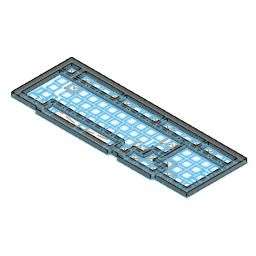
gotta crank v1 (Autodesk Fusion 360 design; units mm, degrees)
Autodesk Fusion 360 part; units mm, degrees
(part 1 of 2)
sketch "plate-2023-07-14T19_23_39.336Z" plane through (0, 0, 0) normal (0, 0, 1) x (1, 0, 0) in component "for my desk"
  arc A0 (50.65, -2.525) -> (50.15, -3.025) centre (50.65, -3.025) ccw
  line L0 (31.1, -3.025) -> (31.1, -16.025)
  line L1 (69.7, -2.525) -> (82.7, -2.525)
  arc A1 (125.5625, -16.525) -> (126.0625, -16.025) centre (125.5625, -16.025) ccw
  line L2 (131.6125, -2.525) -> (144.6125, -2.525)
  line L3 (112.0625, -3.025) -> (112.0625, -16.025)
  line L4 (131.1125, -3.025) -> (131.1125, -16.025)
  arc A2 (82.7, -16.525) -> (83.2, -16.025) centre (82.7, -16.025) ccw
  line L5 (50.65, -16.525) -> (63.65, -16.525)
  arc A3 (101.75, -16.525) -> (102.25, -16.025) centre (101.75, -16.025) ccw
  line L6 (88.25, -3.025) -> (88.25, -16.025)
  line L7 (131.6125, -16.525) -> (144.6125, -16.525)
  line L8 (145.1125, -3.025) -> (145.1125, -16.025)
  arc A4 (145.1125, -3.025) -> (144.6125, -2.525) centre (144.6125, -3.025) ccw
  arc A5 (144.6125, -16.525) -> (145.1125, -16.025) centre (144.6125, -16.025) ccw
  line L9 (150.6625, -16.525) -> (163.6625, -16.525)
  arc A6 (131.1125, -16.025) -> (131.6125, -16.525) centre (131.6125, -16.025) ccw
  arc A7 (150.6625, -2.525) -> (150.1625, -3.025) centre (150.6625, -3.025) ccw
  arc A8 (3.025, -2.525) -> (2.525, -3.025) centre (3.025, -3.025) ccw
  arc A9 (88.25, -16.025) -> (88.75, -16.525) centre (88.75, -16.025) ccw
  arc A10 (63.65, -16.525) -> (64.15, -16.025) centre (63.65, -16.025) ccw
  line L10 (69.2, -3.025) -> (69.2, -16.025)
  arc A11 (64.15, -3.025) -> (63.65, -2.525) centre (63.65, -3.025) ccw
  arc A12 (69.7, -2.525) -> (69.2, -3.025) centre (69.7, -3.025) ccw
  line L11 (126.0625, -3.025) -> (126.0625, -16.025)
  arc A13 (112.0625, -16.025) -> (112.5625, -16.525) centre (112.5625, -16.025) ccw
  arc A14 (131.6125, -2.525) -> (131.1125, -3.025) centre (131.6125, -3.025) ccw
  arc A15 (16.025, -16.525) -> (16.525, -16.025) centre (16.025, -16.025) ccw
  line L12 (150.1625, -3.025) -> (150.1625, -16.025)
  line L13 (31.6, -2.525) -> (44.6, -2.525)
  line L14 (88.75, -2.525) -> (101.75, -2.525)
  arc A16 (44.6, -16.525) -> (45.1, -16.025) centre (44.6, -16.025) ccw
  arc A17 (88.75, -2.525) -> (88.25, -3.025) centre (88.75, -3.025) ccw
  line L15 (50.65, -2.525) -> (63.65, -2.525)
  arc A18 (102.25, -3.025) -> (101.75, -2.525) centre (101.75, -3.025) ccw
  line L16 (112.5625, -16.525) -> (125.5625, -16.525)
  arc A19 (112.5625, -2.525) -> (112.0625, -3.025) centre (112.5625, -3.025) ccw
  arc A20 (126.0625, -3.025) -> (125.5625, -2.525) centre (125.5625, -3.025) ccw
  line L17 (102.25, -3.025) -> (102.25, -16.025)
  arc A21 (163.6625, -16.525) -> (164.1625, -16.025) centre (163.6625, -16.025) ccw
  arc A22 (250.175, -16.025) -> (250.675, -16.525) centre (250.675, -16.025) ccw
  line L18 (250.675, -16.525) -> (263.675, -16.525)
  line L19 (307.0375, -3.025) -> (307.0375, -16.025)
  line L20 (250.175, -3.025) -> (250.175, -16.025)
  line L21 (212.075, -3.025) -> (212.075, -16.025)
  arc A23 (293.0375, -16.025) -> (293.5375, -16.525) centre (293.5375, -16.025) ccw
  line L22 (312.5875, -2.525) -> (325.5875, -2.525)
  line L23 (312.0875, -3.025) -> (312.0875, -16.025)
  arc A24 (206.525, -16.525) -> (207.025, -16.025) centre (206.525, -16.025) ccw
  line L24 (245.125, -3.025) -> (245.125, -16.025)
  line L25 (212.575, -2.525) -> (225.575, -2.525)
  line L26 (287.9875, -3.025) -> (287.9875, -16.025)
  line L27 (169.7125, -2.525) -> (182.7125, -2.525)
  line L28 (2.525, -3.025) -> (2.525, -16.025)
  line L29 (274.4875, -16.525) -> (287.4875, -16.525)
  arc A25 (225.575, -16.525) -> (226.075, -16.025) centre (225.575, -16.025) ccw
  arc A26 (2.525, -16.025) -> (3.025, -16.525) centre (3.025, -16.025) ccw
  line L30 (193.525, -16.525) -> (206.525, -16.525)
  arc A27 (182.7125, -16.525) -> (183.2125, -16.025) centre (182.7125, -16.025) ccw
  line L31 (193.525, -2.525) -> (206.525, -2.525)
  line L32 (183.2125, -3.025) -> (183.2125, -16.025)
  line L33 (231.625, -16.525) -> (244.625, -16.525)
  arc A28 (264.175, -3.025) -> (263.675, -2.525) centre (263.675, -3.025) ccw
  arc A29 (287.4875, -16.525) -> (287.9875, -16.025) centre (287.4875, -16.025) ccw
  arc A30 (245.125, -3.025) -> (244.625, -2.525) centre (244.625, -3.025) ccw
  arc A31 (183.2125, -3.025) -> (182.7125, -2.525) centre (182.7125, -3.025) ccw
  line L34 (69.7, -16.525) -> (82.7, -16.525)
  arc A32 (31.6, -2.525) -> (31.1, -3.025) centre (31.6, -3.025) ccw
  line L35 (231.625, -2.525) -> (244.625, -2.525)
  line L36 (264.175, -3.025) -> (264.175, -16.025)
  line L37 (207.025, -3.025) -> (207.025, -16.025)
  line L38 (293.5375, -2.525) -> (306.5375, -2.525)
  arc A33 (274.4875, -2.525) -> (273.9875, -3.025) centre (274.4875, -3.025) ccw
  arc A34 (212.575, -2.525) -> (212.075, -3.025) centre (212.575, -3.025) ccw
  arc A35 (306.5375, -16.525) -> (307.0375, -16.025) centre (306.5375, -16.025) ccw
  arc A36 (164.1625, -3.025) -> (163.6625, -2.525) centre (163.6625, -3.025) ccw
  arc A37 (193.525, -2.525) -> (193.025, -3.025) centre (193.525, -3.025) ccw
  line L39 (226.075, -3.025) -> (226.075, -16.025)
  arc A38 (307.0375, -3.025) -> (306.5375, -2.525) centre (306.5375, -3.025) ccw
  line L40 (293.5375, -16.525) -> (306.5375, -16.525)
  arc A39 (273.9875, -16.025) -> (274.4875, -16.525) centre (274.4875, -16.025) ccw
  arc A40 (169.2125, -16.025) -> (169.7125, -16.525) centre (169.7125, -16.025) ccw
  arc A41 (150.1625, -16.025) -> (150.6625, -16.525) centre (150.6625, -16.025) ccw
  line L41 (169.2125, -3.025) -> (169.2125, -16.025)
  line L42 (293.0375, -3.025) -> (293.0375, -16.025)
  line L43 (212.575, -16.525) -> (225.575, -16.525)
  arc A42 (287.9875, -3.025) -> (287.4875, -2.525) centre (287.4875, -3.025) ccw
  arc A43 (293.5375, -2.525) -> (293.0375, -3.025) centre (293.5375, -3.025) ccw
  arc A44 (250.675, -2.525) -> (250.175, -3.025) centre (250.675, -3.025) ccw
  arc A45 (120.8, -40.3375) -> (121.3, -39.8375) centre (120.8, -39.8375) ccw
  arc A46 (63.65, -40.3375) -> (64.15, -39.8375) centre (63.65, -39.8375) ccw
  arc A47 (107.8, -26.3375) -> (107.3, -26.8375) centre (107.8, -26.8375) ccw
  arc A48 (244.625, -16.525) -> (245.125, -16.025) centre (244.625, -16.025) ccw
  line L44 (45.1, -26.8375) -> (45.1, -39.8375)
  line L45 (7.2875, -26.8375) -> (7.2875, -39.8375)
  line L46 (69.2, -26.8375) -> (69.2, -39.8375)
  arc A49 (325.5875, -16.525) -> (326.0875, -16.025) centre (325.5875, -16.025) ccw
  arc A50 (312.5875, -2.525) -> (312.0875, -3.025) centre (312.5875, -3.025) ccw
  line L47 (7.7875, -40.3375) -> (20.7875, -40.3375)
  line L48 (31.1, -26.8375) -> (31.1, -39.8375)
  line L49 (145.9, -26.3375) -> (158.9, -26.3375)
  line L50 (145.9, -40.3375) -> (158.9, -40.3375)
  line L51 (145.4, -26.8375) -> (145.4, -39.8375)
  arc A51 (169.7125, -2.525) -> (169.2125, -3.025) centre (169.7125, -3.025) ccw
  line L52 (21.2875, -26.8375) -> (21.2875, -39.8375)
  arc A52 (207.025, -3.025) -> (206.525, -2.525) centre (206.525, -3.025) ccw
  line L53 (50.15, -26.8375) -> (50.15, -39.8375)
  arc A53 (44.6, -40.3375) -> (45.1, -39.8375) centre (44.6, -39.8375) ccw
  line L54 (159.4, -26.8375) -> (159.4, -39.8375)
  arc A54 (126.35, -39.8375) -> (126.85, -40.3375) centre (126.85, -39.8375) ccw
  arc A55 (7.2875, -39.8375) -> (7.7875, -40.3375) centre (7.7875, -39.8375) ccw
  line L55 (64.15, -26.8375) -> (64.15, -39.8375)
  line L56 (273.9875, -3.025) -> (273.9875, -16.025)
  arc A56 (31.6, -26.3375) -> (31.1, -26.8375) centre (31.6, -26.8375) ccw
  arc A57 (88.25, -39.8375) -> (88.75, -40.3375) centre (88.75, -39.8375) ccw
  line L57 (126.35, -26.8375) -> (126.35, -39.8375)
  line L58 (121.3, -26.8375) -> (121.3, -39.8375)
  line L59 (126.85, -26.3375) -> (139.85, -26.3375)
  line L60 (107.8, -26.3375) -> (120.8, -26.3375)
  line L61 (326.0875, -3.025) -> (326.0875, -16.025)
  line L62 (312.5875, -16.525) -> (325.5875, -16.525)
  arc A58 (88.75, -26.3375) -> (88.25, -26.8375) centre (88.75, -26.8375) ccw
  arc A59 (50.15, -39.8375) -> (50.65, -40.3375) centre (50.65, -39.8375) ccw
  arc A60 (69.7, -26.3375) -> (69.2, -26.8375) centre (69.7, -26.8375) ccw
  arc A61 (193.025, -16.025) -> (193.525, -16.525) centre (193.525, -16.025) ccw
  line L63 (140.35, -26.8375) -> (140.35, -39.8375)
  arc A62 (82.7, -40.3375) -> (83.2, -39.8375) centre (82.7, -39.8375) ccw
  line L64 (102.25, -26.8375) -> (102.25, -39.8375)
  arc A63 (101.75, -40.3375) -> (102.25, -39.8375) centre (101.75, -39.8375) ccw
  line L65 (83.2, -26.8375) -> (83.2, -39.8375)
  arc A64 (139.85, -40.3375) -> (140.35, -39.8375) centre (139.85, -39.8375) ccw
  arc A65 (107.3, -39.8375) -> (107.8, -40.3375) centre (107.8, -39.8375) ccw
  arc A66 (20.7875, -40.3375) -> (21.2875, -39.8375) centre (20.7875, -39.8375) ccw
  line L66 (274.4875, -2.525) -> (287.4875, -2.525)
  line L67 (88.75, -40.3375) -> (101.75, -40.3375)
  arc A67 (83.2, -26.8375) -> (82.7, -26.3375) centre (82.7, -26.8375) ccw
  line L68 (250.675, -2.525) -> (263.675, -2.525)
  line L69 (193.025, -3.025) -> (193.025, -16.025)
  arc A68 (212.075, -16.025) -> (212.575, -16.525) centre (212.575, -16.025) ccw
  line L70 (69.7, -26.3375) -> (82.7, -26.3375)
  arc A69 (145.9, -26.3375) -> (145.4, -26.8375) centre (145.9, -26.8375) ccw
  arc A70 (231.625, -2.525) -> (231.125, -3.025) centre (231.625, -3.025) ccw
  line L71 (169.7125, -16.525) -> (182.7125, -16.525)
  arc A71 (226.075, -3.025) -> (225.575, -2.525) centre (225.575, -3.025) ccw
  arc A72 (21.2875, -26.8375) -> (20.7875, -26.3375) centre (20.7875, -26.8375) ccw
  line L72 (231.125, -3.025) -> (231.125, -16.025)
  arc A73 (231.125, -16.025) -> (231.625, -16.525) centre (231.625, -16.025) ccw
  arc A74 (263.675, -16.525) -> (264.175, -16.025) centre (263.675, -16.025) ccw
  arc A75 (69.2, -39.8375) -> (69.7, -40.3375) centre (69.7, -39.8375) ccw
  arc A76 (64.15, -26.8375) -> (63.65, -26.3375) centre (63.65, -26.8375) ccw
  arc A77 (140.35, -26.8375) -> (139.85, -26.3375) centre (139.85, -26.8375) ccw
  line L73 (107.8, -40.3375) -> (120.8, -40.3375)
  arc A78 (121.3, -26.8375) -> (120.8, -26.3375) centre (120.8, -26.8375) ccw
  arc A79 (287.4875, -40.3375) -> (287.9875, -39.8375) centre (287.4875, -39.8375) ccw
  arc A80 (273.9875, -39.8375) -> (274.4875, -40.3375) centre (274.4875, -39.8375) ccw
  line L74 (293.5375, -40.3375) -> (306.5375, -40.3375)
  arc A81 (164.45, -39.8375) -> (164.95, -40.3375) centre (164.95, -39.8375) ccw
  arc A82 (45.1, -26.8375) -> (44.6, -26.3375) centre (44.6, -26.8375) ccw
  line L75 (255.4375, -40.3375) -> (268.4375, -40.3375)
  line L76 (202.55, -26.8375) -> (202.55, -39.8375)
  arc A83 (216.55, -26.8375) -> (216.05, -26.3375) centre (216.05, -26.8375) ccw
  arc A84 (197.5, -26.8375) -> (197, -26.3375) centre (197, -26.8375) ccw
  arc A85 (184, -26.3375) -> (183.5, -26.8375) centre (184, -26.8375) ccw
  line L77 (184, -40.3375) -> (197, -40.3375)
  arc A86 (293.0375, -39.8375) -> (293.5375, -40.3375) centre (293.5375, -39.8375) ccw
  line L78 (274.4875, -40.3375) -> (287.4875, -40.3375)
  arc A87 (268.9375, -26.8375) -> (268.4375, -26.3375) centre (268.4375, -26.8375) ccw
  line L79 (88.75, -26.3375) -> (101.75, -26.3375)
  line L80 (31.6, -40.3375) -> (44.6, -40.3375)
  line L81 (293.0375, -26.8375) -> (293.0375, -39.8375)
  line L82 (126.85, -40.3375) -> (139.85, -40.3375)
  arc A88 (312.0875, -16.025) -> (312.5875, -16.525) centre (312.5875, -16.025) ccw
  line L83 (273.9875, -26.8375) -> (273.9875, -39.8375)
  arc A89 (226.3625, -39.8375) -> (226.8625, -40.3375) centre (226.8625, -39.8375) ccw
  arc A90 (240.3625, -26.8375) -> (239.8625, -26.3375) centre (239.8625, -26.8375) ccw
  arc A91 (183.5, -39.8375) -> (184, -40.3375) centre (184, -39.8375) ccw
  line L84 (50.65, -26.3375) -> (63.65, -26.3375)
  line L85 (88.25, -26.8375) -> (88.25, -39.8375)
  arc A92 (7.7875, -26.3375) -> (7.2875, -26.8375) centre (7.7875, -26.8375) ccw
  arc A93 (255.4375, -26.3375) -> (254.9375, -26.8375) centre (255.4375, -26.8375) ccw
  line L86 (307.0375, -26.8375) -> (307.0375, -39.8375)
  arc A94 (226.8625, -26.3375) -> (226.3625, -26.8375) centre (226.8625, -26.8375) ccw
  line L87 (50.65, -40.3375) -> (63.65, -40.3375)
  arc A95 (306.5375, -40.3375) -> (307.0375, -39.8375) centre (306.5375, -39.8375) ccw
  line L88 (274.4875, -26.3375) -> (287.4875, -26.3375)
  line L89 (7.7875, -26.3375) -> (20.7875, -26.3375)
  arc A96 (145.4, -39.8375) -> (145.9, -40.3375) centre (145.9, -39.8375) ccw
  arc A97 (287.9875, -26.8375) -> (287.4875, -26.3375) centre (287.4875, -26.8375) ccw
  line L90 (293.5375, -26.3375) -> (306.5375, -26.3375)
  arc A98 (307.0375, -26.8375) -> (306.5375, -26.3375) centre (306.5375, -26.8375) ccw
  line L91 (312.5875, -26.3375) -> (325.5875, -26.3375)
  line L92 (216.55, -26.8375) -> (216.55, -39.8375)
  line L93 (312.5875, -40.3375) -> (325.5875, -40.3375)
  line L94 (164.95, -26.3375) -> (177.95, -26.3375)
  line L95 (254.9375, -26.8375) -> (254.9375, -39.8375)
  arc A99 (268.4375, -40.3375) -> (268.9375, -39.8375) centre (268.4375, -39.8375) ccw
  arc A100 (293.5375, -26.3375) -> (293.0375, -26.8375) centre (293.5375, -26.8375) ccw
  line L96 (312.0875, -26.8375) -> (312.0875, -39.8375)
  arc A101 (274.4875, -26.3375) -> (273.9875, -26.8375) centre (274.4875, -26.8375) ccw
  line L97 (31.6, -26.3375) -> (44.6, -26.3375)
  arc A102 (326.0875, -3.025) -> (325.5875, -2.525) centre (325.5875, -3.025) ccw
  arc A103 (31.1, -39.8375) -> (31.6, -40.3375) centre (31.6, -39.8375) ccw
  arc A104 (50.65, -26.3375) -> (50.15, -26.8375) centre (50.65, -26.8375) ccw
  line L98 (107.3, -26.8375) -> (107.3, -39.8375)
  arc A105 (216.05, -40.3375) -> (216.55, -39.8375) centre (216.05, -39.8375) ccw
  line L99 (240.3625, -26.8375) -> (240.3625, -39.8375)
  arc A106 (239.8625, -40.3375) -> (240.3625, -39.8375) centre (239.8625, -39.8375) ccw
  line L100 (197.5, -26.8375) -> (197.5, -39.8375)
  line L101 (178.45, -26.8375) -> (178.45, -39.8375)
  line L102 (268.9375, -26.8375) -> (268.9375, -39.8375)
  line L103 (69.7, -40.3375) -> (82.7, -40.3375)
  arc A107 (102.25, -26.8375) -> (101.75, -26.3375) centre (101.75, -26.8375) ccw
  line L104 (184, -26.3375) -> (197, -26.3375)
  line L105 (203.05, -40.3375) -> (216.05, -40.3375)
  arc A108 (177.95, -40.3375) -> (178.45, -39.8375) centre (177.95, -39.8375) ccw
  line L106 (183.5, -26.8375) -> (183.5, -39.8375)
  arc A109 (126.85, -26.3375) -> (126.35, -26.8375) centre (126.85, -26.8375) ccw
  arc A110 (150.6625, -45.3875) -> (150.1625, -45.8875) centre (150.6625, -45.8875) ccw
  line L107 (49.8625, -45.8875) -> (49.8625, -58.8875)
  arc A111 (10.1687, -45.3875) -> (9.6688, -45.8875) centre (10.1687, -45.8875) ccw
  arc A112 (68.9125, -45.8875) -> (68.4125, -45.3875) centre (68.4125, -45.8875) ccw
  line L108 (164.45, -26.8375) -> (164.45, -39.8375)
  arc A113 (203.05, -26.3375) -> (202.55, -26.8375) centre (203.05, -26.8375) ccw
  line L109 (36.3625, -59.3875) -> (49.3625, -59.3875)
  arc A114 (131.1125, -58.8875) -> (131.6125, -59.3875) centre (131.6125, -58.8875) ccw
  line L110 (112.5625, -45.3875) -> (125.5625, -45.3875)
  arc A115 (178.45, -26.8375) -> (177.95, -26.3375) centre (177.95, -26.8375) ccw
  line L111 (55.4125, -45.3875) -> (68.4125, -45.3875)
  line L112 (131.1125, -45.8875) -> (131.1125, -58.8875)
  arc A116 (158.9, -40.3375) -> (159.4, -39.8375) centre (158.9, -39.8375) ccw
  arc A117 (197, -40.3375) -> (197.5, -39.8375) centre (197, -39.8375) ccw
  line L113 (164.1625, -45.8875) -> (164.1625, -58.8875)
  arc A118 (87.4625, -59.3875) -> (87.9625, -58.8875) centre (87.4625, -58.8875) ccw
  line L114 (73.9625, -45.8875) -> (73.9625, -58.8875)
  line L115 (87.9625, -45.8875) -> (87.9625, -58.8875)
  line L116 (145.1125, -45.8875) -> (145.1125, -58.8875)
  line L117 (68.9125, -45.8875) -> (68.9125, -58.8875)
  arc A119 (107.0125, -45.8875) -> (106.5125, -45.3875) centre (106.5125, -45.8875) ccw
  line L118 (23.6687, -45.8875) -> (23.6687, -58.8875)
  line L119 (74.4625, -45.3875) -> (87.4625, -45.3875)
  line L120 (93.5125, -59.3875) -> (106.5125, -59.3875)
  arc A120 (254.9375, -39.8375) -> (255.4375, -40.3375) centre (255.4375, -39.8375) ccw
  arc A121 (36.3625, -45.3875) -> (35.8625, -45.8875) centre (36.3625, -45.8875) ccw
  line L121 (326.0875, -26.8375) -> (326.0875, -39.8375)
  line L122 (226.8625, -40.3375) -> (239.8625, -40.3375)
  arc A122 (74.4625, -45.3875) -> (73.9625, -45.8875) centre (74.4625, -45.8875) ccw
  arc A123 (144.6125, -59.3875) -> (145.1125, -58.8875) centre (144.6125, -58.8875) ccw
  line L123 (107.0125, -45.8875) -> (107.0125, -58.8875)
  arc A124 (93.5125, -45.3875) -> (93.0125, -45.8875) centre (93.5125, -45.8875) ccw
  line L124 (255.4375, -26.3375) -> (268.4375, -26.3375)
  line L125 (150.1625, -45.8875) -> (150.1625, -58.8875)
  arc A125 (159.4, -26.8375) -> (158.9, -26.3375) centre (158.9, -26.8375) ccw
  line L126 (131.6125, -59.3875) -> (144.6125, -59.3875)
  arc A126 (87.9625, -45.8875) -> (87.4625, -45.3875) centre (87.4625, -45.8875) ccw
  arc A127 (73.9625, -58.8875) -> (74.4625, -59.3875) centre (74.4625, -58.8875) ccw
  line L127 (93.0125, -45.8875) -> (93.0125, -58.8875)
  line L128 (112.5625, -59.3875) -> (125.5625, -59.3875)
  line L129 (203.05, -26.3375) -> (216.05, -26.3375)
  arc A128 (55.4125, -45.3875) -> (54.9125, -45.8875) centre (55.4125, -45.8875) ccw
  line L130 (9.6687, -45.8875) -> (9.6687, -58.8875)
  arc A129 (9.6687, -58.8875) -> (10.1687, -59.3875) centre (10.1687, -58.8875) ccw
  line L131 (35.8625, -45.8875) -> (35.8625, -58.8875)
  arc A130 (93.0125, -58.8875) -> (93.5125, -59.3875) centre (93.5125, -58.8875) ccw
  arc A131 (54.9125, -58.8875) -> (55.4125, -59.3875) centre (55.4125, -58.8875) ccw
  arc A132 (325.5875, -40.3375) -> (326.0875, -39.8375) centre (325.5875, -39.8375) ccw
  line L132 (287.9875, -26.8375) -> (287.9875, -39.8375)
  arc A133 (164.95, -26.3375) -> (164.45, -26.8375) centre (164.95, -26.8375) ccw
  line L133 (10.1687, -45.3875) -> (23.1687, -45.3875)
  line L134 (226.8625, -26.3375) -> (239.8625, -26.3375)
  line L135 (150.6625, -59.3875) -> (163.6625, -59.3875)
  arc A134 (49.8625, -45.8875) -> (49.3625, -45.3875) centre (49.3625, -45.8875) ccw
  arc A135 (312.0875, -39.8375) -> (312.5875, -40.3375) centre (312.5875, -39.8375) ccw
  arc A136 (202.55, -39.8375) -> (203.05, -40.3375) centre (203.05, -39.8375) ccw
  arc A137 (68.4125, -59.3875) -> (68.9125, -58.8875) centre (68.4125, -58.8875) ccw
  line L136 (131.6125, -45.3875) -> (144.6125, -45.3875)
  line L137 (126.0625, -45.8875) -> (126.0625, -58.8875)
  line L138 (164.95, -40.3375) -> (177.95, -40.3375)
  line L139 (55.4125, -59.3875) -> (68.4125, -59.3875)
  arc A138 (312.5875, -26.3375) -> (312.0875, -26.8375) centre (312.5875, -26.8375) ccw
  arc A139 (126.0625, -45.8875) -> (125.5625, -45.3875) centre (125.5625, -45.8875) ccw
  line L140 (226.3625, -26.8375) -> (226.3625, -39.8375)
  line L141 (164.1625, -3.025) -> (164.1625, -16.025)
  line L142 (45.1, -3.025) -> (45.1, -16.025)
  arc A140 (83.2, -3.025) -> (82.7, -2.525) centre (82.7, -3.025) ccw
  line L143 (112.5625, -2.525) -> (125.5625, -2.525)
  arc A141 (16.525, -3.025) -> (16.025, -2.525) centre (16.025, -3.025) ccw
  line L144 (3.025, -16.525) -> (16.025, -16.525)
  arc A142 (31.1, -16.025) -> (31.6, -16.525) centre (31.6, -16.025) ccw
  line L145 (3.025, -2.525) -> (16.025, -2.525)
  line L146 (31.6, -16.525) -> (44.6, -16.525)
  line L147 (16.525, -3.025) -> (16.525, -16.025)
  arc A143 (45.1, -3.025) -> (44.6, -2.525) centre (44.6, -3.025) ccw
  line L148 (150.6625, -2.525) -> (163.6625, -2.525)
  line L149 (50.15, -3.025) -> (50.15, -16.025)
  arc A144 (69.2, -16.025) -> (69.7, -16.525) centre (69.7, -16.025) ccw
  line L150 (64.15, -3.025) -> (64.15, -16.025)
  arc A145 (50.15, -16.025) -> (50.65, -16.525) centre (50.65, -16.025) ccw
  line L151 (88.75, -16.525) -> (101.75, -16.525)
  line L152 (83.2, -3.025) -> (83.2, -16.025)
  line L153 (10.1687, -59.3875) -> (23.1687, -59.3875)
  arc A146 (326.0875, -26.8375) -> (325.5875, -26.3375) centre (325.5875, -26.8375) ccw
  arc A147 (112.5625, -45.3875) -> (112.0625, -45.8875) centre (112.5625, -45.8875) ccw
  arc A148 (23.6687, -45.8875) -> (23.1687, -45.3875) centre (23.1687, -45.8875) ccw
  arc A149 (106.5125, -59.3875) -> (107.0125, -58.8875) centre (106.5125, -58.8875) ccw
  arc A150 (23.1687, -59.3875) -> (23.6687, -58.8875) centre (23.1687, -58.8875) ccw
  arc A151 (131.6125, -45.3875) -> (131.1125, -45.8875) centre (131.6125, -45.8875) ccw
  line L154 (74.4625, -59.3875) -> (87.4625, -59.3875)
  arc A152 (35.8625, -58.8875) -> (36.3625, -59.3875) centre (36.3625, -58.8875) ccw
  line L155 (36.3625, -45.3875) -> (49.3625, -45.3875)
  line L156 (54.9125, -45.8875) -> (54.9125, -58.8875)
  line L157 (93.5125, -45.3875) -> (106.5125, -45.3875)
  arc A153 (49.3625, -59.3875) -> (49.8625, -58.8875) centre (49.3625, -58.8875) ccw
  arc A154 (163.6625, -59.3875) -> (164.1625, -58.8875) centre (163.6625, -58.8875) ccw
  line L158 (307.0375, -45.8875) -> (307.0375, -58.8875)
  arc A155 (241.6567, -46.8875) -> (241.1567, -46.3875) centre (241.1567, -46.8875) ccw
  arc A156 (255.4375, -45.3875) -> (254.9375, -45.8875) centre (255.4375, -45.8875) ccw
  line L159 (274.4875, -45.3875) -> (287.4875, -45.3875)
  arc A157 (274.4875, -45.3875) -> (273.9875, -45.8875) centre (274.4875, -45.8875) ccw
  arc A158 (145.1125, -45.8875) -> (144.6125, -45.3875) centre (144.6125, -45.8875) ccw
  line L160 (219.2188, -45.8875) -> (219.2188, -58.8875)
  arc A159 (211.2808, -46.3875) -> (210.7808, -46.8875) centre (211.2808, -46.8875) ccw
  arc A160 (183.2125, -45.8875) -> (182.7125, -45.3875) centre (182.7125, -45.8875) ccw
  line L161 (235.1568, -61.3875) -> (241.1567, -61.3875)
  arc A161 (293.5375, -45.3875) -> (293.0375, -45.8875) centre (293.5375, -45.8875) ccw
  line L162 (211.2808, -46.3875) -> (217.2808, -46.3875)
  line L163 (268.9375, -45.8875) -> (268.9375, -58.8875)
  arc A162 (112.0625, -58.8875) -> (112.5625, -59.3875) centre (112.5625, -58.8875) ccw
  line L164 (293.0375, -45.8875) -> (293.0375, -58.8875)
  arc A163 (254.9375, -58.8875) -> (255.4375, -59.3875) centre (255.4375, -58.8875) ccw
  arc A164 (232.7188, -59.3875) -> (233.2188, -58.8875) centre (232.7188, -58.8875) ccw
  line L165 (274.4875, -59.3875) -> (287.4875, -59.3875)
  line L166 (188.7625, -45.3875) -> (201.7625, -45.3875)
  arc A165 (219.7188, -45.3875) -> (219.2188, -45.8875) centre (219.7188, -45.8875) ccw
  arc A166 (234.6568, -60.8875) -> (235.1568, -61.3875) centre (235.1568, -60.8875) ccw
  line L167 (112.0625, -45.8875) -> (112.0625, -58.8875)
  line L168 (202.2625, -45.8875) -> (202.2625, -58.8875)
  line L169 (255.4375, -59.3875) -> (268.4375, -59.3875)
  line L170 (150.6625, -45.3875) -> (163.6625, -45.3875)
  line L171 (219.7188, -45.3875) -> (232.7188, -45.3875)
  arc A167 (235.1568, -46.3875) -> (234.6568, -46.8875) centre (235.1568, -46.8875) ccw
  arc A168 (210.7808, -60.8875) -> (211.2808, -61.3875) centre (211.2808, -60.8875) ccw
  line L172 (287.9875, -45.8875) -> (287.9875, -58.8875)
  arc A169 (125.5625, -59.3875) -> (126.0625, -58.8875) centre (125.5625, -58.8875) ccw
  line L173 (325.0875, -70.8505) -> (325.0875, -76.8505)
  arc A170 (201.7625, -59.3875) -> (202.2625, -58.8875) centre (201.7625, -58.8875) ccw
  line L174 (324.5875, -77.3505) -> (310.5875, -77.3505)
  line L175 (241.6567, -46.8875) -> (241.6567, -60.8875)
  arc A171 (287.4875, -59.3875) -> (287.9875, -58.8875) centre (287.4875, -58.8875) ccw
  line L176 (169.2125, -45.8875) -> (169.2125, -58.8875)
  line L177 (312.0875, -55.4125) -> (312.0875, -68.4125)
  arc A172 (45.8875, -64.4375) -> (45.3875, -64.9375) centre (45.8875, -64.9375) ccw
  arc A173 (150.1625, -58.8875) -> (150.6625, -59.3875) centre (150.6625, -58.8875) ccw
  line L178 (183.2125, -45.8875) -> (183.2125, -58.8875)
  arc A174 (169.2125, -58.8875) -> (169.7125, -59.3875) centre (169.7125, -58.8875) ccw
  arc A175 (293.0375, -58.8875) -> (293.5375, -59.3875) centre (293.5375, -58.8875) ccw
  line L179 (217.7808, -46.8875) -> (217.7808, -60.8875)
  line L180 (233.2188, -45.8875) -> (233.2188, -58.8875)
  line L181 (293.5375, -59.3875) -> (306.5375, -59.3875)
  line L182 (310.0875, -70.8505) -> (310.0875, -76.8505)
  line L183 (293.5375, -45.3875) -> (306.5375, -45.3875)
  arc A176 (30.3693, -65.4375) -> (29.8693, -65.9375) centre (30.3693, -65.9375) ccw
  arc A177 (273.9875, -58.8875) -> (274.4875, -59.3875) centre (274.4875, -58.8875) ccw
  arc A178 (325.0875, -46.9745) -> (324.5875, -46.4745) centre (324.5875, -46.9745) ccw
  arc A179 (6.4933, -65.4375) -> (5.9933, -65.9375) centre (6.4933, -65.9375) ccw
  line L184 (169.7125, -59.3875) -> (182.7125, -59.3875)
  line L185 (325.0875, -46.9745) -> (325.0875, -52.9745)
  arc A180 (326.0875, -55.4125) -> (325.5875, -54.9125) centre (325.5875, -55.4125) ccw
  arc A181 (164.1625, -45.8875) -> (163.6625, -45.3875) centre (163.6625, -45.8875) ccw
  line L186 (14.9313, -78.4375) -> (27.9312, -78.4375)
  line L187 (210.7808, -46.8875) -> (210.7808, -60.8875)
  arc A182 (28.4312, -64.9375) -> (27.9312, -64.4375) centre (27.9312, -64.9375) ccw
  line L188 (324.5875, -70.3505) -> (310.5875, -70.3505)
  arc A183 (14.4313, -77.9375) -> (14.9313, -78.4375) centre (14.9313, -77.9375) ccw
  line L189 (254.9375, -45.8875) -> (254.9375, -58.8875)
  line L190 (6.4933, -65.4375) -> (12.4932, -65.4375)
  line L191 (234.6568, -46.8875) -> (234.6568, -60.8875)
  arc A184 (188.7625, -45.3875) -> (188.2625, -45.8875) centre (188.7625, -45.8875) ccw
  arc A185 (202.2625, -45.8875) -> (201.7625, -45.3875) centre (201.7625, -45.8875) ccw
  line L192 (14.9313, -64.4375) -> (27.9312, -64.4375)
  arc A186 (312.0875, -68.4125) -> (312.5875, -68.9125) centre (312.5875, -68.4125) ccw
  arc A187 (188.2625, -58.8875) -> (188.7625, -59.3875) centre (188.7625, -58.8875) ccw
  line L193 (324.5875, -53.4745) -> (310.5875, -53.4745)
  line L194 (235.1568, -46.3875) -> (241.1567, -46.3875)
  line L195 (188.2625, -45.8875) -> (188.2625, -58.8875)
  line L196 (273.9875, -45.8875) -> (273.9875, -58.8875)
  arc A188 (268.4375, -59.3875) -> (268.9375, -58.8875) centre (268.4375, -58.8875) ccw
  line L197 (45.8875, -64.4375) -> (58.8875, -64.4375)
  arc A189 (217.7808, -46.8875) -> (217.2808, -46.3875) centre (217.2808, -46.8875) ccw
  arc A190 (310.5875, -46.4745) -> (310.0875, -46.9745) centre (310.5875, -46.9745) ccw
  arc A191 (324.5875, -77.3505) -> (325.0875, -76.8505) centre (324.5875, -76.8505) ccw
  line L198 (325.5875, -54.9125) -> (312.5875, -54.9125)
  arc A192 (169.7125, -45.3875) -> (169.2125, -45.8875) centre (169.7125, -45.8875) ccw
  line L199 (219.7188, -59.3875) -> (232.7188, -59.3875)
  line L200 (211.2808, -61.3875) -> (217.2808, -61.3875)
  arc A193 (268.9375, -45.8875) -> (268.4375, -45.3875) centre (268.4375, -45.8875) ccw
  arc A194 (233.2188, -45.8875) -> (232.7188, -45.3875) centre (232.7188, -45.8875) ccw
  arc A195 (241.1567, -61.3875) -> (241.6567, -60.8875) centre (241.1567, -60.8875) ccw
  arc A196 (287.9875, -45.8875) -> (287.4875, -45.3875) centre (287.4875, -45.8875) ccw
  line L201 (255.4375, -45.3875) -> (268.4375, -45.3875)
  line L202 (188.7625, -59.3875) -> (201.7625, -59.3875)
  line L203 (169.7125, -45.3875) -> (182.7125, -45.3875)
  arc A197 (219.2188, -58.8875) -> (219.7188, -59.3875) centre (219.7188, -58.8875) ccw
  arc A198 (217.2808, -61.3875) -> (217.7808, -60.8875) centre (217.2808, -60.8875) ccw
  arc A199 (182.7125, -59.3875) -> (183.2125, -58.8875) centre (182.7125, -58.8875) ccw
  line L204 (28.4312, -64.9375) -> (28.4313, -77.9375)
  line L205 (326.0875, -55.4125) -> (326.0875, -68.4125)
  line L206 (325.5875, -68.9125) -> (312.5875, -68.9125)
  line L207 (216.55, -64.9375) -> (216.55, -77.9375)
  arc A200 (83.9875, -64.4375) -> (83.4875, -64.9375) centre (83.9875, -64.9375) ccw
  arc A201 (310.5875, -70.3505) -> (310.0875, -70.8505) centre (310.5875, -70.8505) ccw
  line L208 (122.0875, -64.4375) -> (135.0875, -64.4375)
  arc A202 (306.5375, -59.3875) -> (307.0375, -58.8875) centre (306.5375, -58.8875) ccw
  line L209 (140.6375, -64.9375) -> (140.6375, -77.9375)
  arc A203 (121.5875, -77.9375) -> (122.0875, -78.4375) centre (122.0875, -77.9375) ccw
  arc A204 (324.5875, -53.4745) -> (325.0875, -52.9745) centre (324.5875, -52.9745) ccw
  line L210 (29.8693, -65.9375) -> (29.8693, -79.9375)
  arc A205 (45.3875, -77.9375) -> (45.8875, -78.4375) centre (45.8875, -77.9375) ccw
  arc A206 (29.8693, -79.9375) -> (30.3693, -80.4375) centre (30.3693, -79.9375) ccw
  arc A207 (325.0875, -70.8505) -> (324.5875, -70.3505) centre (324.5875, -70.8505) ccw
  line L211 (36.8693, -65.9375) -> (36.8693, -79.9375)
  line L212 (116.5375, -64.9375) -> (116.5375, -77.9375)
  line L213 (203.05, -78.4375) -> (216.05, -78.4375)
  arc A208 (173.6875, -64.9375) -> (173.1875, -64.4375) centre (173.1875, -64.9375) ccw
  line L214 (14.4313, -64.9375) -> (14.4313, -77.9375)
  line L215 (78.4375, -64.9375) -> (78.4375, -77.9375)
  arc A209 (12.9932, -65.9375) -> (12.4932, -65.4375) centre (12.4932, -65.9375) ccw
  arc A210 (192.7375, -64.9375) -> (192.2375, -64.4375) centre (192.2375, -64.9375) ccw
  line L216 (255.4375, -64.4375) -> (268.4375, -64.4375)
  arc A211 (160.1875, -64.4375) -> (159.6875, -64.9375) centre (160.1875, -64.9375) ccw
  line L217 (179.2375, -64.4375) -> (192.2375, -64.4375)
  arc A212 (102.5375, -77.9375) -> (103.0375, -78.4375) centre (103.0375, -77.9375) ccw
  line L218 (141.1375, -78.4375) -> (154.1375, -78.4375)
  arc A213 (179.2375, -64.4375) -> (178.7375, -64.9375) centre (179.2375, -64.9375) ccw
  arc A214 (83.4875, -77.9375) -> (83.9875, -78.4375) centre (83.9875, -77.9375) ccw
  line L219 (203.05, -64.4375) -> (216.05, -64.4375)
  arc A215 (36.3693, -80.4375) -> (36.8693, -79.9375) centre (36.3693, -79.9375) ccw
  arc A216 (216.05, -78.4375) -> (216.55, -77.9375) centre (216.05, -77.9375) ccw
  line L220 (121.5875, -64.9375) -> (121.5875, -77.9375)
  arc A217 (36.8693, -65.9375) -> (36.3693, -65.4375) centre (36.3693, -65.9375) ccw
  arc A218 (192.2375, -78.4375) -> (192.7375, -77.9375) centre (192.2375, -77.9375) ccw
  arc A219 (310.0875, -76.8505) -> (310.5875, -77.3505) centre (310.5875, -76.8505) ccw
  line L221 (45.8875, -78.4375) -> (58.8875, -78.4375)
  arc A220 (5.9932, -79.9375) -> (6.4933, -80.4375) centre (6.4933, -79.9375) ccw
  arc A221 (312.5875, -54.9125) -> (312.0875, -55.4125) centre (312.5875, -55.4125) ccw
  arc A222 (58.8875, -78.4375) -> (59.3875, -77.9375) centre (58.8875, -77.9375) ccw
  arc A223 (307.0375, -45.8875) -> (306.5375, -45.3875) centre (306.5375, -45.8875) ccw
  arc A224 (14.9313, -64.4375) -> (14.4313, -64.9375) centre (14.9313, -64.9375) ccw
  line L222 (45.3875, -64.9375) -> (45.3875, -77.9375)
  arc A225 (27.9312, -78.4375) -> (28.4312, -77.9375) centre (27.9312, -77.9375) ccw
  line L223 (64.4375, -64.9375) -> (64.4375, -77.9375)
  arc A226 (12.4932, -80.4375) -> (12.9933, -79.9375) centre (12.4932, -79.9375) ccw
  line L224 (83.4875, -64.9375) -> (83.4875, -77.9375)
  line L225 (64.9375, -78.4375) -> (77.9375, -78.4375)
  arc A227 (64.9375, -64.4375) -> (64.4375, -64.9375) centre (64.9375, -64.9375) ccw
  line L226 (202.55, -64.9375) -> (202.55, -77.9375)
  line L227 (64.9375, -64.4375) -> (77.9375, -64.4375)
  line L228 (310.0875, -46.9745) -> (310.0875, -52.9745)
  line L229 (5.9932, -65.9375) -> (5.9932, -79.9375)
  line L230 (30.3693, -80.4375) -> (36.3693, -80.4375)
  line L231 (324.5875, -46.4745) -> (310.5875, -46.4745)
  line L232 (160.1875, -64.4375) -> (173.1875, -64.4375)
  arc A228 (59.3875, -64.9375) -> (58.8875, -64.4375) centre (58.8875, -64.9375) ccw
  arc A229 (310.0875, -52.9745) -> (310.5875, -53.4745) centre (310.5875, -52.9745) ccw
  line L233 (97.4875, -64.9375) -> (97.4875, -77.9375)
  line L234 (159.6875, -64.9375) -> (159.6875, -77.9375)
  line L235 (6.4933, -80.4375) -> (12.4932, -80.4375)
  line L236 (12.9932, -65.9375) -> (12.9932, -79.9375)
  line L237 (30.3693, -65.4375) -> (36.3693, -65.4375)
  arc A230 (325.5875, -68.9125) -> (326.0875, -68.4125) centre (325.5875, -68.4125) ccw
  line L238 (59.3875, -64.9375) -> (59.3875, -77.9375)
  arc A231 (141.1375, -64.4375) -> (140.6375, -64.9375) centre (141.1375, -64.9375) ccw
  arc A232 (244.625, -83.2) -> (245.125, -82.7) centre (244.625, -82.7) ccw
  arc A233 (231.125, -82.7) -> (231.625, -83.2) centre (231.625, -82.7) ccw
  arc A234 (78.4375, -64.9375) -> (77.9375, -64.4375) centre (77.9375, -64.9375) ccw
  arc A235 (64.4375, -77.9375) -> (64.9375, -78.4375) centre (64.9375, -77.9375) ccw
  line L239 (178.7375, -64.9375) -> (178.7375, -77.9375)
  arc A236 (274.4875, -83.4875) -> (273.9875, -83.9875) centre (274.4875, -83.9875) ccw
  line L240 (268.9375, -64.9375) -> (268.9375, -77.9375)
  arc A237 (18.4062, -97.4875) -> (18.9063, -96.9875) centre (18.4062, -96.9875) ccw
  line L241 (26.8375, -97.4875) -> (39.8375, -97.4875)
  arc A238 (293.5375, -64.4375) -> (293.0375, -64.9375) centre (293.5375, -64.9375) ccw
  arc A239 (255.4375, -64.4375) -> (254.9375, -64.9375) centre (255.4375, -64.9375) ccw
  arc A240 (103.0375, -64.4375) -> (102.5375, -64.9375) centre (103.0375, -64.9375) ccw
  line L242 (173.6875, -64.9375) -> (173.6875, -77.9375)
  arc A241 (122.0875, -64.4375) -> (121.5875, -64.9375) centre (122.0875, -64.9375) ccw
  arc A242 (203.05, -64.4375) -> (202.55, -64.9375) centre (203.05, -64.9375) ccw
  arc A243 (173.1875, -78.4375) -> (173.6875, -77.9375) centre (173.1875, -77.9375) ccw
  line L243 (255.4375, -78.4375) -> (268.4375, -78.4375)
  arc A244 (154.6375, -64.9375) -> (154.1375, -64.4375) centre (154.1375, -64.9375) ccw
  arc A245 (273.9875, -77.9375) -> (274.4875, -78.4375) centre (274.4875, -77.9375) ccw
  arc A246 (159.6875, -77.9375) -> (160.1875, -78.4375) centre (160.1875, -77.9375) ccw
  arc A247 (140.6375, -77.9375) -> (141.1375, -78.4375) centre (141.1375, -77.9375) ccw
  line L244 (135.5875, -64.9375) -> (135.5875, -77.9375)
  line L245 (160.1875, -78.4375) -> (173.1875, -78.4375)
  line L246 (274.4875, -78.4375) -> (287.4875, -78.4375)
  line L247 (103.0375, -78.4375) -> (116.0375, -78.4375)
  line L248 (40.3375, -83.9875) -> (40.3375, -96.9875)
  line L249 (83.9875, -64.4375) -> (96.9875, -64.4375)
  line L250 (274.4875, -64.4375) -> (287.4875, -64.4375)
  arc A248 (178.7375, -77.9375) -> (179.2375, -78.4375) centre (179.2375, -77.9375) ccw
  arc A249 (96.9875, -78.4375) -> (97.4875, -77.9375) centre (96.9875, -77.9375) ccw
  line L251 (103.0375, -64.4375) -> (116.0375, -64.4375)
  line L252 (293.5375, -78.4375) -> (306.5375, -78.4375)
  arc A250 (268.4375, -78.4375) -> (268.9375, -77.9375) centre (268.4375, -77.9375) ccw
  arc A251 (245.125, -69.7) -> (244.625, -69.2) centre (244.625, -69.7) ccw
  arc A252 (307.0375, -64.9375) -> (306.5375, -64.4375) centre (306.5375, -64.9375) ccw
  arc A253 (202.2625, -83.9875) -> (201.7625, -83.4875) centre (201.7625, -83.9875) ccw
  line L253 (231.625, -83.2) -> (244.625, -83.2)
  line L254 (26.8375, -83.4875) -> (39.8375, -83.4875)
  arc A254 (116.5375, -64.9375) -> (116.0375, -64.4375) centre (116.0375, -64.9375) ccw
  arc A255 (274.4875, -64.4375) -> (273.9875, -64.9375) centre (274.4875, -64.9375) ccw
  arc A256 (202.55, -77.9375) -> (203.05, -78.4375) centre (203.05, -77.9375) ccw
  line L255 (83.9875, -78.4375) -> (96.9875, -78.4375)
  line L256 (122.0875, -78.4375) -> (135.0875, -78.4375)
  arc A257 (216.55, -64.9375) -> (216.05, -64.4375) centre (216.05, -64.9375) ccw
  line L257 (141.1375, -64.4375) -> (154.1375, -64.4375)
  arc A258 (77.9375, -78.4375) -> (78.4375, -77.9375) centre (77.9375, -77.9375) ccw
  arc A259 (135.0875, -78.4375) -> (135.5875, -77.9375) centre (135.0875, -77.9375) ccw
  line L258 (274.4875, -83.4875) -> (287.4875, -83.4875)
  line L259 (192.7375, -64.9375) -> (192.7375, -77.9375)
  line L260 (179.2375, -78.4375) -> (192.2375, -78.4375)
  arc A260 (306.5375, -78.4375) -> (307.0375, -77.9375) centre (306.5375, -77.9375) ccw
  arc A261 (116.0375, -78.4375) -> (116.5375, -77.9375) centre (116.0375, -77.9375) ccw
  arc A262 (97.4875, -64.9375) -> (96.9875, -64.4375) centre (96.9875, -64.9375) ccw
  arc A263 (26.3375, -96.9875) -> (26.8375, -97.4875) centre (26.8375, -96.9875) ccw
  arc A264 (287.4875, -97.4875) -> (287.9875, -96.9875) centre (287.4875, -96.9875) ccw
  line L261 (26.3375, -83.9875) -> (26.3375, -96.9875)
  line L262 (273.9875, -64.9375) -> (273.9875, -77.9375)
  line L263 (102.5375, -64.9375) -> (102.5375, -77.9375)
  arc A265 (135.5875, -64.9375) -> (135.0875, -64.4375) centre (135.0875, -64.9375) ccw
  arc A266 (154.1375, -78.4375) -> (154.6375, -77.9375) centre (154.1375, -77.9375) ccw
  line L264 (154.6375, -64.9375) -> (154.6375, -77.9375)
  line L265 (254.9375, -64.9375) -> (254.9375, -77.9375)
  line L266 (231.625, -69.2) -> (244.625, -69.2)
  arc A267 (201.7625, -97.4875) -> (202.2625, -96.9875) centre (201.7625, -96.9875) ccw
  line L267 (293.5375, -64.4375) -> (306.5375, -64.4375)
  line L268 (250.175, -88.75) -> (250.175, -101.75)
  arc A268 (254.9375, -77.9375) -> (255.4375, -78.4375) centre (255.4375, -77.9375) ccw
  arc A269 (39.8375, -97.4875) -> (40.3375, -96.9875) centre (39.8375, -96.9875) ccw
  line L269 (264.175, -88.75) -> (264.175, -101.75)
  arc A270 (231.625, -69.2) -> (231.125, -69.7) centre (231.625, -69.7) ccw
  arc A271 (293.5375, -83.4875) -> (293.0375, -83.9875) centre (293.5375, -83.9875) ccw
  line L270 (293.5375, -83.4875) -> (306.5375, -83.4875)
  arc A272 (60.15, -104.25) -> (60.65, -103.75) centre (60.15, -103.75) ccw
  arc A273 (174.95, -89.75) -> (174.45, -89.25) centre (174.45, -89.75) ccw
  line L271 (307.0375, -64.9375) -> (307.0375, -77.9375)
  line L272 (231.125, -88.75) -> (231.125, -101.75)
  arc A274 (231.625, -88.25) -> (231.125, -88.75) centre (231.625, -88.75) ccw
  arc A275 (188.2625, -96.9875) -> (188.7625, -97.4875) centre (188.7625, -96.9875) ccw
  arc A276 (231.125, -101.75) -> (231.625, -102.25) centre (231.625, -101.75) ccw
  arc A277 (174.45, -104.25) -> (174.95, -103.75) centre (174.45, -103.75) ccw
  arc A278 (226.075, -88.75) -> (225.575, -88.25) centre (225.575, -88.75) ccw
  arc A279 (245.125, -88.75) -> (244.625, -88.25) centre (244.625, -88.75) ccw
  line L273 (188.2625, -83.9875) -> (188.2625, -96.9875)
  line L274 (312.5875, -97.4875) -> (325.5875, -97.4875)
  arc A280 (121.3, -88.75) -> (120.8, -88.25) centre (120.8, -88.75) ccw
  line L275 (5.4062, -83.4875) -> (18.4063, -83.4875)
  line L276 (18.9062, -83.9875) -> (18.9063, -96.9875)
  arc A281 (120.8, -102.25) -> (121.3, -101.75) centre (120.8, -101.75) ccw
  line L277 (60.65, -89.75) -> (60.65, -103.75)
  line L278 (212.575, -102.25) -> (225.575, -102.25)
  line L279 (121.3, -88.75) -> (121.3, -101.75)
  arc A282 (53.65, -103.75) -> (54.15, -104.25) centre (54.15, -103.75) ccw
  line L280 (231.625, -102.25) -> (244.625, -102.25)
  arc A283 (264.175, -88.75) -> (263.675, -88.25) centre (263.675, -88.75) ccw
  line L281 (293.0375, -64.9375) -> (293.0375, -77.9375)
  line L282 (312.0875, -83.9875) -> (312.0875, -96.9875)
  arc A284 (250.175, -101.75) -> (250.675, -102.25) centre (250.675, -101.75) ccw
  line L283 (307.0375, -83.9875) -> (307.0375, -96.9875)
  arc A285 (273.9875, -96.9875) -> (274.4875, -97.4875) centre (274.4875, -96.9875) ccw
  line L284 (293.0375, -83.9875) -> (293.0375, -96.9875)
  arc A286 (40.3375, -83.9875) -> (39.8375, -83.4875) centre (39.8375, -83.9875) ccw
  line L285 (293.5375, -97.4875) -> (306.5375, -97.4875)
  line L286 (287.9875, -64.9375) -> (287.9875, -77.9375)
  arc A287 (293.0375, -77.9375) -> (293.5375, -78.4375) centre (293.5375, -77.9375) ccw
  line L287 (245.125, -69.7) -> (245.125, -82.7)
  line L288 (202.2625, -83.9875) -> (202.2625, -96.9875)
  arc A288 (287.9875, -64.9375) -> (287.4875, -64.4375) centre (287.4875, -64.9375) ccw
  line L289 (188.7625, -97.4875) -> (201.7625, -97.4875)
  line L290 (107.8, -88.25) -> (120.8, -88.25)
  line L291 (212.075, -88.75) -> (212.075, -101.75)
  line L292 (287.9875, -83.9875) -> (287.9875, -96.9875)
  arc A289 (244.625, -102.25) -> (245.125, -101.75) centre (244.625, -101.75) ccw
  line L293 (273.9875, -83.9875) -> (273.9875, -96.9875)
  line L294 (188.7625, -83.4875) -> (201.7625, -83.4875)
  line L295 (231.125, -69.7) -> (231.125, -82.7)
  arc A290 (287.4875, -78.4375) -> (287.9875, -77.9375) centre (287.4875, -77.9375) ccw
  line L296 (4.9062, -83.9875) -> (4.9062, -96.9875)
  line L297 (274.4875, -97.4875) -> (287.4875, -97.4875)
  arc A291 (18.9062, -83.9875) -> (18.4062, -83.4875) centre (18.4062, -83.9875) ccw
  arc A292 (287.9875, -83.9875) -> (287.4875, -83.4875) centre (287.4875, -83.9875) ccw
  arc A293 (5.4062, -83.4875) -> (4.9062, -83.9875) centre (5.4062, -83.9875) ccw
  arc A294 (26.8375, -83.4875) -> (26.3375, -83.9875) centre (26.8375, -83.9875) ccw
  arc A295 (4.9062, -96.9875) -> (5.4062, -97.4875) centre (5.4062, -96.9875) ccw
  arc A296 (268.9375, -64.9375) -> (268.4375, -64.4375) centre (268.4375, -64.9375) ccw
  arc A297 (312.5875, -83.4875) -> (312.0875, -83.9875) centre (312.5875, -83.9875) ccw
  arc A298 (188.7625, -83.4875) -> (188.2625, -83.9875) centre (188.7625, -83.9875) ccw
  arc A299 (307.0375, -83.9875) -> (306.5375, -83.4875) centre (306.5375, -83.9875) ccw
  line L298 (5.4062, -97.4875) -> (18.4063, -97.4875)
  arc A300 (225.575, -102.25) -> (226.075, -101.75) centre (225.575, -101.75) ccw
  arc A301 (212.075, -101.75) -> (212.575, -102.25) centre (212.575, -101.75) ccw
  line L299 (168.45, -104.25) -> (174.45, -104.25)
  line L300 (107.8, -102.25) -> (120.8, -102.25)
  line L301 (0, -100.0125) -> (0, 0)
  line L302 (250.675, -102.25) -> (263.675, -102.25)
  arc A302 (250.675, -88.25) -> (250.175, -88.75) centre (250.675, -88.75) ccw
  line L303 (312.5875, -83.4875) -> (325.5875, -83.4875)
  arc A303 (212.575, -88.25) -> (212.075, -88.75) centre (212.575, -88.75) ccw
  line L304 (53.65, -89.75) -> (53.65, -103.75)
  arc A304 (326.0875, -83.9875) -> (325.5875, -83.4875) centre (325.5875, -83.9875) ccw
  line L305 (328.6125, -100.0125) -> (328.6125, 0)
  line L306 (245.125, -88.75) -> (245.125, -101.75)
  arc A305 (312.0875, -96.9875) -> (312.5875, -97.4875) centre (312.5875, -96.9875) ccw
  arc A306 (306.5375, -97.4875) -> (307.0375, -96.9875) centre (306.5375, -96.9875) ccw
  arc A307 (107.8, -88.25) -> (107.3, -88.75) centre (107.8, -88.75) ccw
  line L307 (250.675, -88.25) -> (263.675, -88.25)
  line L308 (326.0875, -83.9875) -> (326.0875, -96.9875)
  line L309 (212.575, -88.25) -> (225.575, -88.25)
  line L310 (226.075, -88.75) -> (226.075, -101.75)
  arc A308 (60.65, -89.75) -> (60.15, -89.25) centre (60.15, -89.75) ccw
  arc A309 (325.5875, -97.4875) -> (326.0875, -96.9875) centre (325.5875, -96.9875) ccw
  line L311 (231.625, -88.25) -> (244.625, -88.25)
  arc A310 (107.3, -101.75) -> (107.8, -102.25) centre (107.8, -101.75) ccw
  line L312 (168.45, -89.25) -> (174.45, -89.25)
  line L313 (0, 0) -> (328.6125, 0)
  line L314 (54.15, -89.25) -> (60.15, -89.25)
  arc A311 (168.45, -89.25) -> (167.95, -89.75) centre (168.45, -89.75) ccw
  arc A312 (293.0375, -96.9875) -> (293.5375, -97.4875) centre (293.5375, -96.9875) ccw
  line L315 (54.15, -104.25) -> (60.15, -104.25)
  line L316 (174.95, -89.75) -> (174.95, -103.75)
  line L317 (167.95, -89.75) -> (167.95, -103.75)
  arc A313 (263.675, -102.25) -> (264.175, -101.75) centre (263.675, -101.75) ccw
  arc A314 (167.95, -103.75) -> (168.45, -104.25) centre (168.45, -103.75) ccw
  line L318 (107.3, -88.75) -> (107.3, -101.75)
  arc A315 (54.15, -89.25) -> (53.65, -89.75) centre (54.15, -89.75) ccw
  line L319 (0, 0) -> (19.05, 0)
  line L320 (19.05, 0) -> (19.05, -19.05)
  line L321 (19.05, -19.05) -> (0, -19.05)
  line L322 (0, -19.05) -> (0, 0)
  line L323 (0, 0) -> (19.05, -19.05) construction
  line L324 (19.05, 0) -> (0, -19.05) construction
  line L325 (47.625, 0) -> (28.575, 0)
  line L326 (28.575, 0) -> (28.575, -19.05)
  line L327 (28.575, -19.05) -> (47.625, -19.05)
  line L328 (47.625, -19.05) -> (47.625, 0) construction
  line L329 (47.625, 0) -> (28.575, -19.05) construction
  line L330 (28.575, 0) -> (47.625, -19.05) construction
  line L331 (47.625, -23.8125) -> (28.575, -23.8125)
  line L332 (28.575, -23.8125) -> (28.575, -42.8625) construction
  line L333 (28.575, -42.8625) -> (47.625, -42.8625) construction
  line L334 (47.625, -42.8625) -> (47.625, -23.8125) construction
  line L335 (47.625, -23.8125) -> (28.575, -42.8625) construction
  line L336 (28.575, -23.8125) -> (47.625, -42.8625) construction
  line L337 (85.725, 0) -> (104.775, 0)
  line L338 (104.775, 0) -> (104.775, -19.05)
  line L339 (104.775, -19.05) -> (85.725, -19.05)
  line L340 (85.725, -19.05) -> (85.725, 0) construction
  line L341 (85.725, 0) -> (104.775, -19.05) construction
  line L342 (104.775, 0) -> (85.725, -19.05) construction
  line L343 (128.5875, 0) -> (109.5375, 0)
  line L344 (109.5375, 0) -> (109.5375, -19.05)
  line L345 (109.5375, -19.05) -> (128.5875, -19.05)
  line L346 (128.5875, -19.05) -> (128.5875, 0) construction
  line L347 (128.5875, 0) -> (109.5375, -19.05) construction
  line L348 (109.5375, 0) -> (128.5875, -19.05) construction
  line L349 (185.7375, 0) -> (166.6875, 0)
  line L350 (166.6875, 0) -> (166.6875, -19.05) construction
  line L351 (166.6875, -19.05) -> (185.7375, -19.05)
  line L352 (185.7375, -19.05) -> (185.7375, 0)
  line L353 (185.7375, 0) -> (166.6875, -19.05) construction
  line L354 (166.6875, 0) -> (185.7375, -19.05) construction
  line L355 (209.55, 0) -> (190.5, 0)
  line L356 (190.5, 0) -> (190.5, -19.05)
  line L357 (190.5, -19.05) -> (209.55, -19.05)
  line L358 (209.55, -19.05) -> (209.55, 0) construction
  line L359 (209.55, 0) -> (190.5, -19.05) construction
  line L360 (190.5, 0) -> (209.55, -19.05) construction
  line L361 (290.5125, 0) -> (271.4625, 0)
  line L362 (271.4625, 0) -> (271.4625, -19.05)
  line L363 (271.4625, -19.05) -> (290.5125, -19.05)
  line L364 (290.5125, -19.05) -> (290.5125, 0) construction
  line L365 (290.5125, 0) -> (271.4625, -19.05) construction
  line L366 (271.4625, 0) -> (290.5125, -19.05) construction
  line L367 (266.7, 0) -> (247.65, 0)
  line L368 (247.65, 0) -> (247.65, -19.05) construction
  line L369 (247.65, -19.05) -> (266.7, -19.05)
  line L370 (266.7, -19.05) -> (266.7, 0)
  line L371 (266.7, 0) -> (247.65, -19.05) construction
  line L372 (247.65, 0) -> (266.7, -19.05) construction
  line L373 (266.7, -104.775) -> (247.65, -104.775)
  line L374 (247.65, -104.775) -> (247.65, -85.725) construction
  line L375 (247.65, -85.725) -> (266.7, -85.725)
  line L376 (266.7, -85.725) -> (266.7, -104.775)
  line L377 (266.7, -104.775) -> (247.65, -85.725) construction
  line L378 (247.65, -104.775) -> (266.7, -85.725) construction
  line L379 (247.65, -85.725) -> (228.6, -85.725) construction
  line L380 (228.6, -85.725) -> (228.6, -66.675)
  line L381 (228.6, -66.675) -> (247.65, -66.675)
  line L382 (247.65, -66.675) -> (247.65, -85.725)
  line L383 (247.65, -85.725) -> (228.6, -66.675) construction
  line L384 (228.6, -85.725) -> (247.65, -66.675) construction
  line L385 (228.6, -85.725) -> (209.55, -85.725)
  line L386 (209.55, -85.725) -> (209.55, -104.775)
  line L387 (209.55, -104.775) -> (228.6, -104.775)
  line L388 (228.6, -104.775) -> (228.6, -85.725) construction
  line L389 (228.6, -85.725) -> (209.55, -104.775) construction
  line L390 (209.55, -85.725) -> (228.6, -104.775) construction
  line L391 (204.7875, -100.0125) -> (185.7375, -100.0125)
  line L392 (185.7375, -100.0125) -> (185.7375, -80.9625)
  line L393 (185.7375, -80.9625) -> (204.7875, -80.9625) construction
  line L394 (204.7875, -80.9625) -> (204.7875, -100.0125)
  line L395 (204.7875, -100.0125) -> (185.7375, -80.9625) construction
  line L396 (185.7375, -100.0125) -> (204.7875, -80.9625) construction
  line L397 (180.975, -104.775) -> (47.625, -104.775)
  line L398 (47.625, -104.775) -> (47.625, -85.725)
  line L399 (47.625, -85.725) -> (180.975, -85.725)
  line L400 (180.975, -85.725) -> (180.975, -104.775)
  line L401 (180.975, -104.775) -> (47.625, -85.725) construction
  line L402 (47.625, -104.775) -> (180.975, -85.725) construction
  line L403 (42.8625, -100.0125) -> (23.8125, -100.0125)
  line L404 (42.8625, -80.9625) -> (42.8625, -100.0125)
  line L405 (42.8625, -100.0125) -> (23.8125, -80.9625) construction
  line L406 (23.8125, -100.0125) -> (42.8625, -80.9625) construction
  line L407 (290.5125, -80.9625) -> (271.4625, -80.9625) construction
  line L408 (271.4625, -80.9625) -> (271.4625, -100.0125)
  line L409 (271.4625, -100.0125) -> (290.5125, -100.0125)
  line L410 (290.5125, -100.0125) -> (290.5125, -80.9625) construction
  line L411 (290.5125, -80.9625) -> (271.4625, -100.0125) construction
  line L412 (271.4625, -80.9625) -> (290.5125, -100.0125) construction
  line L413 (271.4625, -80.9625) -> (252.4125, -80.9625)
  line L414 (252.4125, -80.9625) -> (252.4125, -61.9125)
  line L415 (252.4125, -61.9125) -> (271.4625, -61.9125) construction
  line L416 (271.4625, -61.9125) -> (271.4625, -80.9625) construction
  line L417 (271.4625, -80.9625) -> (252.4125, -61.9125) construction
  line L418 (252.4125, -80.9625) -> (271.4625, -61.9125) construction
  line L419 (28.575, -23.8125) -> (0, -23.8125)
  line L420 (195.2625, -80.9625) -> (223.8375, -80.9625)
  line L421 (223.8375, -80.9625) -> (223.8375, -61.9125)
  line L422 (223.8375, -61.9125) -> (195.2625, -61.9125) construction
  line L423 (195.2625, -61.9125) -> (195.2625, -80.9625) construction
  line L424 (195.2625, -80.9625) -> (223.8375, -61.9125) construction
  line L425 (223.8375, -80.9625) -> (195.2625, -61.9125) construction
  line L426 (247.65, -42.8625) -> (219.075, -42.8625) construction
  line L427 (219.075, -42.8625) -> (219.075, -23.8125) construction
  line L428 (219.075, -23.8125) -> (247.65, -23.8125)